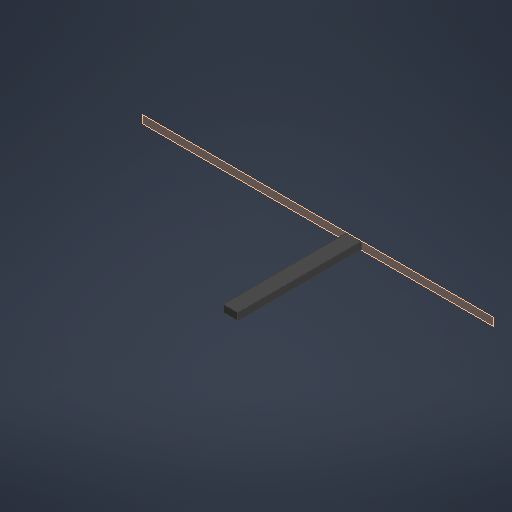
# Autodesk Inventor part: Rename
Saved by Autodesk Inventor 2027 (Build 310192000, 192)
## iProperties
Created: 2026-08-07
Part Number: Rename
Material: Generic
Document SubType Name: Modeling
Designer: lucas
Density: 1 g/cm^3
Appearance: Default
Author: lucas
Autodesk Inventor part; units mm, degrees
ref_plane "YZ Plane" through (0, 0, 0) normal (1, 0, 0) x (0, 1, 0)
ref_plane "XZ Plane" through (0, 0, 0) normal (0, 1, 0) x (-1, 0, 0)
ref_plane "XY Plane" through (0, 0, 0) normal (0, 0, 1) x (1, 0, 0)
ref_plane "Work Plane1" through (0, 0, 0) normal (0, 0, 1) x (1, 0, 0)
sketch "Sketch1" plane through (0, 0, 0) normal (0, 0, 1) x (1, 0, 0)
  line L0 (2235.2, 0) -> (0, 0) projected
  line L1 (0, 0) -> (0, 50.8) projected
  line L2 (2235.2, 50.8) -> (0, 50.8) projected
  line L3 (2235.2, 0) -> (2235.2, 50.8) projected
  line L4 (1320.8, 0) -> (1320.8, 50.8) projected
  line L5 (1422.4, 0) -> (1320.8, 0) projected
  line L6 (1422.4, 50.8) -> (1422.4, 0) projected
  line L7 (2235.2, 50.8) -> (0, 50.8) projected
  line L8 (1422.4, 0) -> (1320.8, 0)
  line L9 (1320.8, 0) -> (1320.8, 50.8)
  line L10 (1320.8, 50.8) -> (1422.4, 50.8)
  line L11 (1422.4, 50.8) -> (1422.4, 0)
  constraints: 8 end point, 2 parallel, 1 horizontal, 1 perpendicular
extrude "Extrusion1" add sketch "Sketch1" along normal blind 863.6 contours L0 L4 L2 L6
body "Solid1"
